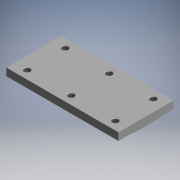
# Autodesk Inventor part: TBCKsupport_plate-MA5150_r
Saved by Autodesk Inventor 2017.3 (Build 213256000, 256)
## iProperties
Part Number: TBCKsupport_plate-MA5150_r
Material: Generic
Catalog Web Link: www.cadenas.de
Description: TBCK_XL, TBCK_L, TBCK_H, TBCK_S3M, TBCK_S5M, TBCK_S8M, TBCK_MA3, TBCK_MA5, TBCK_MA8, TBCK_T5, TBCK_T10, TBCK_AT5, TBCK_AT10_rack-Metal Fittings for Timing Belts - Press Prevention Type
Vendor: MISUMI
Document SubType Name: Modeling
Designer: partserver
Manufacturer: MISUMI
Mass: 9.53131 g
Surface Area: 57.7291 cm^2
Volume: 9.53131 cm^3
Density: 1 g/cm^3
Appearance: PSOLRGB-192-192-192
Category: PARTsolutions
Company: MISUMI
Title: TBCKsupport_plate-MA5150
Author: Cadenas PARTsolutions
Comments: Metal Fittings for Timing Belts - Press Prevention Type
PSOL_IDENT_0: {$CADENAS_DATA\23d-libs\misumi\metric\48_timing_belts\tbck_rack.prj},316 {VTYP=3D},{NB=TBCKsupport_p
PSOL_IDENT_1: late-MA5150_r},{LINA=TBCKsupport_plate-MA5150},{NN=TBCK_XL, TBCK_L, TBCK_H, TBCK_S3M, TBCK_S5M, TBCK
PSOL_IDENT_2: _S8M, TBCK_MA3, TBCK_MA5, TBCK_MA8, TBCK_T5, TBCK_T10, TBCK_AT5, TBCK_AT10_rack},{DATE=08.06.2021 08
PSOL_IDENT_3: :28:56},{GEOMDATE=14.02.2020 07:54:32},{VERSION=},{LINEID=120},{WBVAR=BNW},{WBNUMERIC=}  {NB=TBCKsup
PSOL_IDENT_4: port_plate-MA5150_r},{LINA=TBCKsupport_plate-MA5150},{KT=DUMMY},{PN=TBCKsupport_plate-MA5150},{TYPE=
PSOL_IDENT_5: TBCK},{MAT=A6N01-T5},{ST=Clear Adonize},{AC=Hexagon Socket Head Cap Screw},{TB=MA5},{BNW=150},{BNW1='
PSOL_IDENT_6: 100','100','150','150','250','250'},{W=15.0},{A=65},{B=32},{T1=6},{T2=5.5},{T3=2.90},{HH=1.70},{L=51
PSOL_IDENT_7: },{P=22},{M=M4},{M1=4},{DD=4.5},{AB=M4-10},{AB1=10},{NMH=6},{ANGLE=0.000},{LR=0.0000},{PITCH=5.000},
PSOL_IDENT_8: {RR=0.500},{RA=0.000},{LL=3.250},{NT=0}
NB: TBCKsupport_plate-MA5150_r
NN: TBCK_XL, TBCK_L, TBCK_H, TBCK_S3M, TBCK_S5M, TBCK_S8M, TBCK_MA3, TBCK_MA5, TBCK_MA8, TBCK_T5, TBCK_T10, TBCK_AT5, TBCK_AT10_rack
NT: 0
NBSYN: $PN._r
LINA: TBCKsupport_plate-MA5150
CATALOG: Misumi
PN: TBCKsupport_plate-MA5150
MAT: A6N01-T5
ST: Clear Adonize
AC: Hexagon Socket Head Cap Screw
TB: MA5
BNW: 150
W: 15
A: 65
B: 32
T1: 6
T2: 5.5
T3: 2.9
HH: 1.7
L: 51
P: 22
M: M4
DD: 4.5
AB: M4-10
NMH: 6
SUPPLIER: MISUMI
ARTICLENO: TBCKsupport_plate-MA5150_r
BOMINFO: TBCKsupport_plate-MA5150
CREATOR: CADENAS GmbH
Autodesk Inventor part; units mm, degrees
sketch "Sketch_1" plane through (0, 0, 0) normal (0, 0, 1) x (1, 0, 0)
  line L0 (0, 16) -> (0, -16)
  line L1 (0, -16) -> (65, -16)
  line L2 (65, -16) -> (65, 16)
  line L3 (65, 16) -> (0, 16)
  constraints: 8 end point
extrude "Extrusion1" add sketch "Sketch_1" along normal blind 6
sketch "Sketch_2" plane through (0, 0, 0) normal (1, 0, 0) x (0, 1, 0)
  line L0 (16, 6) -> (7.5, 6)
  line L1 (7.5, 6) -> (7.5, 4.3)
  line L2 (7.5, 4.3) -> (16, 4.3)
  line L3 (16, 4.3) -> (16, 6)
  constraints: 8 end point
extrude "Extrusion2" cut sketch "Sketch_2" along normal blind 65
sketch "Sketch_3" plane through (0, 0, 0) normal (1, 0, 0) x (0, 1, 0)
  line L0 (-7.5, 6) -> (-16, 6)
  line L1 (-16, 6) -> (-16, 4.3)
  line L2 (-16, 4.3) -> (-7.5, 4.3)
  line L3 (-7.5, 4.3) -> (-7.5, 6)
  constraints: 8 end point
extrude "Extrusion3" cut sketch "Sketch_3" along normal blind 65
sketch "Sketch_4" plane through (0, 11, 0) normal (0, 1, 0) x (1, 0, 0)
  line L0 (7, 0) -> (7, -4.3)
  line L1 (7, -4.3) -> (5, -4.3)
  line L2 (5, -4.3) -> (5.379, -3.921)
  line L3 (5.379, -3.921) -> (5.379, -0.379)
  line L4 (5.379, -0.379) -> (5, 0)
  line L5 (5, 0) -> (7, 0)
  line L6 (7, 0) -> (7, -4.3)
  constraints: 14 end point
revolve "Revolution1" cut sketch "Sketch_4" angle 360 about axis through (7, 11, 0) along (0, 0, -1)
thread "Thread1" size "M4x0.7" class "6H" standard "ISO Metric profile" full length
pattern_linear "Rectangular Pattern1" count 3 spacing 25.5 along (1, 0, 0) count 2 spacing 22 along (0, -1, 0) of "Revolution1"
sketch "Sketch_8" plane through (0, -7.5, 0) normal (0, 1, 0) x (1, 0, 0)
  line L0 (0, -4.725) -> (0, -10.3)
  line L1 (0, -10.3) -> (65, -10.3)
  line L2 (65, -10.3) -> (65, -4.725)
  arc A0 (63.8551, -4.3) -> (65, -4.725) centre (65, -2.9703) ccw
  arc A1 (63.8551, -4.3) -> (63.3805, -5.8116) centre (66.625, -6) ccw
  arc A2 (63.1808, -6) -> (63.3805, -5.8116) centre (63.1808, -5.8) ccw
  line L3 (63.1808, -6) -> (61.8192, -6)
  arc A3 (61.6195, -5.8116) -> (61.8192, -6) centre (61.8192, -5.8) ccw
  arc A4 (61.6195, -5.8116) -> (61.1449, -4.3) centre (58.375, -6) ccw
  arc A5 (58.8551, -4.3) -> (61.1449, -4.3) centre (60, -2.9703) ccw
  arc A6 (58.8551, -4.3) -> (58.3805, -5.8116) centre (61.625, -6) ccw
  arc A7 (58.1808, -6) -> (58.3805, -5.8116) centre (58.1808, -5.8) ccw
  line L4 (58.1808, -6) -> (56.8192, -6)
  arc A8 (56.6195, -5.8116) -> (56.8192, -6) centre (56.8192, -5.8) ccw
  arc A9 (56.6195, -5.8116) -> (56.1449, -4.3) centre (53.375, -6) ccw
  arc A10 (53.8551, -4.3) -> (56.1449, -4.3) centre (55, -2.9703) ccw
  arc A11 (53.8551, -4.3) -> (53.3805, -5.8116) centre (56.625, -6) ccw
  arc A12 (53.1808, -6) -> (53.3805, -5.8116) centre (53.1808, -5.8) ccw
  line L5 (53.1808, -6) -> (51.8192, -6)
  arc A13 (51.6195, -5.8116) -> (51.8192, -6) centre (51.8192, -5.8) ccw
  arc A14 (51.6195, -5.8116) -> (51.1449, -4.3) centre (48.375, -6) ccw
  arc A15 (48.8551, -4.3) -> (51.1449, -4.3) centre (50, -2.9703) ccw
  arc A16 (48.8551, -4.3) -> (48.3805, -5.8116) centre (51.625, -6) ccw
  arc A17 (48.1808, -6) -> (48.3805, -5.8116) centre (48.1808, -5.8) ccw
  line L6 (48.1808, -6) -> (46.8192, -6)
  arc A18 (46.6195, -5.8116) -> (46.8192, -6) centre (46.8192, -5.8) ccw
  arc A19 (46.6195, -5.8116) -> (46.1449, -4.3) centre (43.375, -6) ccw
  arc A20 (43.8551, -4.3) -> (46.1449, -4.3) centre (45, -2.9703) ccw
  arc A21 (43.8551, -4.3) -> (43.3805, -5.8116) centre (46.625, -6) ccw
  arc A22 (43.1808, -6) -> (43.3805, -5.8116) centre (43.1808, -5.8) ccw
  line L7 (43.1808, -6) -> (41.8192, -6)
  arc A23 (41.6195, -5.8116) -> (41.8192, -6) centre (41.8192, -5.8) ccw
  arc A24 (41.6195, -5.8116) -> (41.1449, -4.3) centre (38.375, -6) ccw
  arc A25 (38.8551, -4.3) -> (41.1449, -4.3) centre (40, -2.9703) ccw
  arc A26 (38.8551, -4.3) -> (38.3805, -5.8116) centre (41.625, -6) ccw
  arc A27 (38.1808, -6) -> (38.3805, -5.8116) centre (38.1808, -5.8) ccw
  line L8 (38.1808, -6) -> (36.8192, -6)
  arc A28 (36.6195, -5.8116) -> (36.8192, -6) centre (36.8192, -5.8) ccw
  arc A29 (36.6195, -5.8116) -> (36.1449, -4.3) centre (33.375, -6) ccw
  arc A30 (33.8551, -4.3) -> (36.1449, -4.3) centre (35, -2.9703) ccw
  arc A31 (33.8551, -4.3) -> (33.3805, -5.8116) centre (36.625, -6) ccw
  arc A32 (33.1808, -6) -> (33.3805, -5.8116) centre (33.1808, -5.8) ccw
  line L9 (33.1808, -6) -> (31.8192, -6)
  arc A33 (31.6195, -5.8116) -> (31.8192, -6) centre (31.8192, -5.8) ccw
  arc A34 (31.6195, -5.8116) -> (31.1449, -4.3) centre (28.375, -6) ccw
  arc A35 (28.8551, -4.3) -> (31.1449, -4.3) centre (30, -2.9703) ccw
  arc A36 (28.8551, -4.3) -> (28.3805, -5.8116) centre (31.625, -6) ccw
  arc A37 (28.1808, -6) -> (28.3805, -5.8116) centre (28.1808, -5.8) ccw
  line L10 (28.1808, -6) -> (26.8192, -6)
  arc A38 (26.6195, -5.8116) -> (26.8192, -6) centre (26.8192, -5.8) ccw
  arc A39 (26.6195, -5.8116) -> (26.1449, -4.3) centre (23.375, -6) ccw
  arc A40 (23.8551, -4.3) -> (26.1449, -4.3) centre (25, -2.9703) ccw
  arc A41 (23.8551, -4.3) -> (23.3805, -5.8116) centre (26.625, -6) ccw
  arc A42 (23.1808, -6) -> (23.3805, -5.8116) centre (23.1808, -5.8) ccw
  line L11 (23.1808, -6) -> (21.8192, -6)
  arc A43 (21.6195, -5.8116) -> (21.8192, -6) centre (21.8192, -5.8) ccw
  arc A44 (21.6195, -5.8116) -> (21.1449, -4.3) centre (18.375, -6) ccw
  arc A45 (18.8551, -4.3) -> (21.1449, -4.3) centre (20, -2.9703) ccw
  arc A46 (18.8551, -4.3) -> (18.3805, -5.8116) centre (21.625, -6) ccw
  arc A47 (18.1808, -6) -> (18.3805, -5.8116) centre (18.1808, -5.8) ccw
  line L12 (18.1808, -6) -> (16.8192, -6)
  arc A48 (16.6195, -5.8116) -> (16.8192, -6) centre (16.8192, -5.8) ccw
  arc A49 (16.6195, -5.8116) -> (16.1449, -4.3) centre (13.375, -6) ccw
  arc A50 (13.8551, -4.3) -> (16.1449, -4.3) centre (15, -2.9703) ccw
  arc A51 (13.8551, -4.3) -> (13.3805, -5.8116) centre (16.625, -6) ccw
  arc A52 (13.1808, -6) -> (13.3805, -5.8116) centre (13.1808, -5.8) ccw
  line L13 (13.1808, -6) -> (11.8192, -6)
  arc A53 (11.6195, -5.8116) -> (11.8192, -6) centre (11.8192, -5.8) ccw
  arc A54 (11.6195, -5.8116) -> (11.1449, -4.3) centre (8.375, -6) ccw
  arc A55 (8.8551, -4.3) -> (11.1449, -4.3) centre (10, -2.9703) ccw
  arc A56 (8.8551, -4.3) -> (8.3805, -5.8116) centre (11.625, -6) ccw
  arc A57 (8.1808, -6) -> (8.3805, -5.8116) centre (8.1808, -5.8) ccw
  line L14 (8.1808, -6) -> (6.8192, -6)
  arc A58 (6.6195, -5.8116) -> (6.8192, -6) centre (6.8192, -5.8) ccw
  arc A59 (6.6195, -5.8116) -> (6.1449, -4.3) centre (3.375, -6) ccw
  arc A60 (3.8551, -4.3) -> (6.1449, -4.3) centre (5, -2.9703) ccw
  arc A61 (3.8551, -4.3) -> (3.3805, -5.8116) centre (6.625, -6) ccw
  arc A62 (3.1808, -6) -> (3.3805, -5.8116) centre (3.1808, -5.8) ccw
  line L15 (3.1808, -6) -> (1.8192, -6)
  arc A63 (1.6195, -5.8116) -> (1.8192, -6) centre (1.8192, -5.8) ccw
  arc A64 (1.6195, -5.8116) -> (1.1449, -4.3) centre (-1.625, -6) ccw
  arc A65 (0, -4.725) -> (1.1449, -4.3) centre (0, -2.9703) ccw
  constraints: 132 point on circle, 66 centre point, 32 end point
extrude "Extrusion4" cut sketch "Sketch_8" along normal blind 15
ref_plane "tbck_XY" through (0, 0, 4.3) normal (0, 0, -1) x (1, 0, 0)
ref_plane "tbck_YZ" through (0, 0, 4.3) normal (1, 0, 0) x (0, -1, 0)
ref_plane "tbck_ZX" through (0, 0, 4.3) normal (0, -1, 0) x (0, 0, -1)
body "Solid1"
